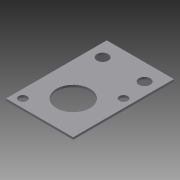
# Autodesk Inventor part: launcher_hinge
Saved by Autodesk Inventor 2013 (Build 170138000, 138)
## iProperties
Created: 2013-07-25
Part Number: launcher_hinge
Material: Generic
Document SubType Name: Modeling
Designer: dkboone
Density: 1 g/cm^3
Author: dkboone
Autodesk Inventor part; units mm, degrees
ref_plane "YZ Plane" through (0, 0, 0) normal (1, 0, 0) x (0, 1, 0)
ref_plane "XZ Plane" through (0, 0, 0) normal (0, 1, 0) x (-1, 0, 0)
ref_plane "XY Plane" through (0, 0, 0) normal (0, 0, 1) x (1, 0, 0)
sketch "Sketch1" plane through (0, 0, 0) normal (0, 1, 0) x (-1, 0, 0)
  line L0 (-12.7, 25.4) -> (12.7, 25.4)
  line L1 (12.7, 25.4) -> (12.7, -12.7)
  line L2 (12.7, -12.7) -> (-12.7, -12.7)
  line L3 (-12.7, -12.7) -> (-12.7, 25.4)
  line L4 (-12.7, 0) -> (12.7, 0) construction
  circle A0 centre (0, 12.7) radius 6.35
  circle A1 centre (9.525, 22.225) radius 1.5875
  circle A2 centre (-9.525, 3.175) radius 1.5875
  circle A3 centre (-7.9375, -6.35) radius 2.1526
  circle A4 centre (7.9375, -6.35) radius 2.1526
  point P0 (0, 0)
  point P1 (0, 0)
  dimension "d0" = 12.7
  dimension "d2" = 25.4
  dimension "d3" = 25.4
  dimension "d4" = 12.7
  dimension "d5" = 3.175
  dimension "d6" = 3.175
  dimension "d7" = 4.3053
  dimension "d8" = 4.3053
  dimension "d9" = 3.175
  dimension "d10" = 3.175
  dimension "d11" = 3.175
  dimension "d12" = 3.175
  dimension "d13" = 12.7
  dimension "d14" = 12.7
  dimension "d15" = 6.35
  dimension "d16" = 6.35
  dimension "d17" = 15.875
  dimension "d18" = 4.7625
  constraints: 10 end point, 5 centre point, 2 parallel, 2 perpendicular, 2 point on line, 1 coincident, 1 horizontal, 1 midpoint
  measures "d0" distance between parallel lines of L4 L2
  measures "d2" distance of L0.start L0.end
  measures "d3" distance between parallel lines of L0 L4
  measures "d4" diameter of A0
  measures "d5" diameter of A2
  measures "d6" diameter of A1
  measures "d7" diameter of A3
  measures "d8" diameter of A4
  measures "d9" distance from line of A2.centre L4
  measures "d10" distance from line of L3 A2.centre
  measures "d11" distance from line of L0 A1.centre
  measures "d12" distance from line of L1 A1.centre
  measures "d13" distance from line of L4 A0.centre
  measures "d14" distance from line of L1 A0.centre
  measures "d15" distance from line of L4 A3.centre
  measures "d16" distance from line of L4 A4.centre
  measures "d17" distance of A4.centre A3.centre
  measures "d18" distance from line of L1 A4.centre
extrude "Extrusion1" add sketch "Sketch1" along normal blind 0.7874
equation "\"d15\" = 0.5 * d0"
equation "\"d16\" = d15"
equation "\"d18\" = -0.5 * d17 + 0.5 * d2"
body "Solid1"
